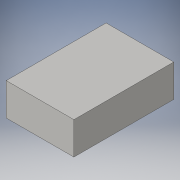
# Autodesk Inventor part: DB9Plug
Saved by Autodesk Inventor 2016 (Build 200138000, 138)
## iProperties
Created: 2016-08-11
Part Number: DB9Plug
Material: Generic
Document SubType Name: Modeling
Designer: jfixelle
Density: 1 g/cm^3
Appearance: Default
Author: jfixelle
Autodesk Inventor part; units mm, degrees
ref_plane "YZ Plane" through (0, 0, 0) normal (1, 0, 0) x (0, 1, 0)
ref_plane "XZ Plane" through (0, 0, 0) normal (0, 1, 0) x (-1, 0, 0)
ref_plane "XY Plane" through (0, 0, 0) normal (0, 0, 1) x (1, 0, 0)
sketch "Sketch1" plane through (0, 0, 0) normal (0, 1, 0) x (-1, 0, 0)
  line L0 (23.174, 28.7337) -> (-10.226, 28.7337)
  line L1 (-10.226, 28.7337) -> (-10.226, -20.5663)
  line L2 (-10.226, -20.5663) -> (23.174, -20.5663)
  line L3 (23.174, -20.5663) -> (23.174, 28.7337)
  point P0 (0, 0)
  dimension "d0" = 49.3
  dimension "d1" = 33.4
  constraints: 8 end point, 2 parallel, 1 horizontal, 1 perpendicular
  measures "d0" distance of L2.end L0.start
  measures "d1" distance of L0.start L0.end
extrude "Extrusion1" add sketch "Sketch1" along normal blind 16
body "Solid1"
